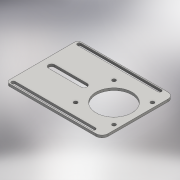
# Autodesk Inventor part: X-motor-holder
Saved by Autodesk Inventor 2016 (Build 200138000, 138)
## iProperties
Created: 2015-05-16
Part Number: X-motor-holder
Material: Generic
Document SubType Name: Modeling
Designer: as
Density: 1 g/cm^3
Appearance: Default
Mass: 6.945 g
Surface Area: 84.6953 cm^2
Volume: 6.945 cm^3
Author: as
Autodesk Inventor part; units mm, degrees
ref_plane "YZ Plane" through (0, 0, 0) normal (1, 0, 0) x (0, 1, 0)
ref_plane "XZ Plane" through (0, 0, 0) normal (0, 1, 0) x (-1, 0, 0)
ref_plane "XY Plane" through (0, 0, 0) normal (0, 0, 1) x (1, 0, 0)
sketch "Sketch1" plane through (0, 0, 0) normal (0, 0, 1) x (1, 0, 0)
  circle A0 centre (0, 0) radius 15 projected
  circle A1 centre (16, 16) radius 1.5 projected
  circle A2 centre (-16, 16) radius 1.5 projected
  circle A3 centre (-16, -16) radius 1.5 projected
  circle A4 centre (16, -16) radius 1.5 projected
  line L0 (20, -18) -> (20, 18) projected
  line L1 (18, 20) -> (-18, 20) projected
  line L2 (-60.0198, 26.9978) -> (-59.9853, -20.0189)
  line L3 (-18, -20) -> (18, -20) projected
  line L4 (-57.0198, 30) -> (-15.022, 30)
  line L5 (-14.978, -30) -> (-56.9802, -30)
  line L6 (-59.9802, -27.0022) -> (-60.0198, 26.9978)
  line L7 (-57.9798, -27.5) -> (12.0202, -27.5) construction
  line L8 (-56.4798, -29) -> (10.5202, -29)
  line L9 (10.5202, -26) -> (-56.4798, -26)
  arc A5 (-56.4798, -26) -> (-56.4798, -29) centre (-56.4798, -27.5) ccw
  arc A6 (10.5202, -29) -> (10.5202, -26) centre (10.5202, -27.5) ccw
  arc A7 (-59.9802, -27.0022) -> (-56.9802, -30) centre (-56.9802, -27) ccw
  arc A8 (-57.0198, 30) -> (-60.0198, 26.9978) centre (-57.0198, 27) ccw
  line L10 (-58.0202, 27.5) -> (11.9798, 27.5) construction
  line L11 (-56.5202, 26) -> (10.4798, 26)
  line L12 (10.4798, 29) -> (-56.5202, 29)
  arc A9 (-56.5202, 29) -> (-56.5202, 26) centre (-56.5202, 27.5) ccw
  arc A10 (10.4798, 26) -> (10.4798, 29) centre (10.4798, 27.5) ccw
  line L13 (20, -18) -> (20, 18)
  line L14 (-14.978, -30) -> (20, -30)
  line L15 (20, -30) -> (20, -18)
  line L16 (20, -30) -> (-56.9802, -30)
  line L17 (-60.0198, -29) -> (-60.0198, 27)
  line L18 (-57.0198, 30) -> (20, 30)
  line L19 (20, 30) -> (20, -30)
  point P0 (0, 0)
  point P1 (-60.0198, 26.9811)
  point P2 (-59.978, -30)
  point P3 (-22.9798, -27.5)
  point P4 (-23.0202, 27.5)
  dimension "d11" = 70
  dimension "d12" = 3
  dimension "d13" = 2.5
  dimension "d15" = 3.5
  dimension "d16" = 3
  dimension "d17" = 3
  dimension "d18" = 3
  dimension "d19" = 70
  dimension "d21" = 3.5
  dimension "d26" = 30
  dimension "d27" = 60
  dimension "d28" = 2.5
  dimension "d29" = 45
  dimension "d30" = 45
  dimension "d31" = 60
  dimension "d32" = 79.9853
  dimension "d33" = 80.0198
  constraints: 38 end point, 17 point on circle, 13 tangent, 9 point on line, 6 centre point, 5 parallel, 4 horizontal, 3 perpendicular, 2 midpoint, 1 vertical
  measures "d11" distance of L7.start L7.end
  measures "d12" diameter of A6
  measures "d13" distance between parallel lines of L5 L7
  measures "d15" distance from line of L6 A5.centre
  measures "d16" radius of A7
  measures "d17" radius of A8
  measures "d18" diameter of A10
  measures "d19" distance of L10.start L10.end
  measures "d21" distance from line of L2 A9.centre
  measures "d26" distance from line of point (0, 0) L5
  measures "d27" distance between parallel lines of L4 L5
  measures "d28" distance from line of L4 point (-23.02, 27.5)
  measures "d29" distance from line of L4.end L2
  measures "d30" distance from line of L2 L5.start
  measures "d31" distance from line of point (0, 0) L6
  measures "d32" distance from line of L2.end L0
  measures "d33" distance from line of point (-60.02, 26.981) L0
extrude "Extrusion1" add sketch "Sketch1" along normal blind 2
fillet "Fillet1" radius 5 2 edges at (20, -30, 1) (20, 30, 1)
sketch "Sketch4" plane through (0, 0, 2) normal (0, 0, 1) x (1, 0, 0)
  line L0 (-22.4, -0.0183) -> (-54.6, -0.0183) construction
  line L1 (-25, 2.5817) -> (-52, 2.5817)
  line L2 (-52, -2.6183) -> (-25, -2.6183)
  arc A0 (-25, -2.6183) -> (-25, 2.5817) centre (-25, -0.0183) ccw
  arc A1 (-52, 2.5817) -> (-52, -2.6183) centre (-52, -0.0183) ccw
  circle A2 centre (0, 0) radius 15 projected
  line L3 (-60.0198, 26.9978) -> (-59.9802, -27.0022) projected
  point P0 (0, 0)
  point P1 (-38.5, -0.0183)
  dimension "d34" = 5.2
  dimension "d35" = 25
  dimension "d36" = 8
  constraints: 8 end point, 6 point on circle, 4 tangent, 2 centre point, 2 point on line, 1 horizontal, 1 midpoint, 1 parallel
  measures "d34" diameter of A1
  measures "d35" distance of A2.centre A0.centre
  measures "d36" distance from line of L3 A1.centre
extrude "Extrusion2" cut sketch "Sketch4" against normal through all contours A0 L2 A1 L1
equation "\"d18\" = d12"
equation "\"d19\" = d11"
equation "\"d21\" = d15"
equation "\"d26\" = 0.5 * d27"
equation "\"d30\" = d29"
body "Solid1"
